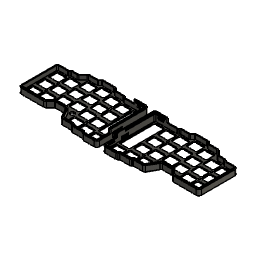
mriya-bumper-fdm-v1.04 (Autodesk Fusion 360 design; units mm, degrees)
Autodesk Fusion 360 part; units mm, degrees
(part 1 of 2)
sketch "mriya" plane through (0, 0, 0) normal (0, 0, 1) x (1, 0, 0)
  line L0 (-101.0213, 15.6719) -> (-94.7787, 21.9145) construction
  line L1 (-26.4858, 1.079) -> (-27.6142, 2.2074) construction
  line L2 (-138.1, 14.7932) -> (-103.1426, 14.7932) construction
  line L3 (-44.0716, 2.7932) -> (-29.0284, 2.7932) construction
  line L4 (-8.6, 0.4932) -> (-25.0716, 0.4932) construction
  line L5 (-64.4741, 6.1094) -> (-72.7517, 20.7608) construction
  line L6 (-45.4858, 3.379) -> (-46.6142, 4.5074) construction
  line L7 (-122.6142, 71.579) -> (-121.4858, 72.7074) construction
  line L8 (-101.0716, 81.2932) -> (-87.2284, 81.2932) construction
  line L9 (-138.1, 70.9932) -> (-124.0284, 70.9932) construction
  line L10 (-92.6574, 22.7932) -> (-76.2344, 22.7932) construction
  line L11 (-48.0284, 5.0932) -> (-62.7328, 5.0932) construction
  line L12 (-82.0716, 84.7932) -> (-64.7284, 84.7932) construction
  line L13 (-58.5716, 80.2932) -> (-45.7284, 80.2932) construction
  line L14 (-24.1, 19.4932) -> (-7.1, 19.4932) construction
  line L15 (-25.6, 20.9932) -> (-25.6, 77.9932) construction
  line L16 (-83.4858, 84.2074) -> (-85.8142, 81.879) construction
  line L17 (-63.3142, 84.2074) -> (-59.9858, 80.879) construction
  line L18 (-139.6, 69.4932) -> (-139.6, 16.2932) construction
  line L19 (-43.1858, 78.579) -> (-44.3142, 79.7074) construction
  line L20 (-99.4, 40.3932) -> (-99.4, 27.9932) construction
  line L21 (-98.6, 41.1932) -> (-86.2, 41.1932) construction
  line L22 (-98.6, 27.1932) -> (-86.2, 27.1932) construction
  line L23 (-85.4, 40.3932) -> (-85.4, 27.9932) construction
  line L24 (-42.4, 56.0932) -> (-42.4, 43.6932) construction
  line L25 (-41.6, 56.8932) -> (-29.2, 56.8932) construction
  line L26 (-41.6, 42.8932) -> (-29.2, 42.8932) construction
  line L27 (-28.4, 56.0932) -> (-28.4, 43.6932) construction
  line L28 (-61.4, 58.3932) -> (-61.4, 45.9932) construction
  line L29 (-60.6, 59.1932) -> (-48.2, 59.1932) construction
  line L30 (-60.6, 45.1932) -> (-48.2, 45.1932) construction
  line L31 (-47.4, 58.3932) -> (-47.4, 45.9932) construction
  line L32 (-137.4, 68.0932) -> (-137.4, 55.6932) construction
  line L33 (-136.6, 68.8932) -> (-124.2, 68.8932) construction
  line L34 (-136.6, 54.8932) -> (-124.2, 54.8932) construction
  line L35 (-123.4, 68.0932) -> (-123.4, 55.6932) construction
  line L36 (-61.4, 39.3932) -> (-61.4, 26.9932) construction
  line L37 (-60.6, 40.1932) -> (-48.2, 40.1932) construction
  line L38 (-60.6, 26.1932) -> (-48.2, 26.1932) construction
  line L39 (-47.4, 39.3932) -> (-47.4, 26.9932) construction
  line L40 (-42.4, 18.0932) -> (-42.4, 5.6932) construction
  line L41 (-41.6, 18.8932) -> (-29.2, 18.8932) construction
  line L42 (-41.6, 4.8932) -> (-29.2, 4.8932) construction
  line L43 (-28.4, 18.0932) -> (-28.4, 5.6932) construction
  line L44 (-23.4, 15.7932) -> (-23.4, 3.3932) construction
  line L45 (-22.6, 16.5932) -> (-10.2, 16.5932) construction
  line L46 (-22.6, 2.5932) -> (-10.2, 2.5932) construction
  line L47 (-9.4, 15.7932) -> (-9.4, 3.3932) construction
  line L48 (-137.4, 49.0932) -> (-137.4, 36.6932) construction
  line L49 (-136.6, 49.8932) -> (-124.2, 49.8932) construction
  line L50 (-136.6, 35.8932) -> (-124.2, 35.8932) construction
  line L51 (-123.4, 49.0932) -> (-123.4, 36.6932) construction
  line L52 (-118.4, 51.3932) -> (-118.4, 38.9932) construction
  line L53 (-117.6, 52.1932) -> (-105.2, 52.1932) construction
  line L54 (-117.6, 38.1932) -> (-105.2, 38.1932) construction
  line L55 (-104.4, 51.3932) -> (-104.4, 38.9932) construction
  line L56 (-137.4, 30.0932) -> (-137.4, 17.6932) construction
  line L57 (-136.6, 30.8932) -> (-124.2, 30.8932) construction
  line L58 (-136.6, 16.8932) -> (-124.2, 16.8932) construction
  line L59 (-123.4, 30.0932) -> (-123.4, 17.6932) construction
  line L60 (-61.4, 20.3932) -> (-61.4, 7.9932) construction
  line L61 (-60.6, 21.1932) -> (-48.2, 21.1932) construction
  line L62 (-60.6, 7.1932) -> (-48.2, 7.1932) construction
  line L63 (-47.4, 20.3932) -> (-47.4, 7.9932) construction
  line L64 (-80.4, 43.8932) -> (-80.4, 31.4932) construction
  line L65 (-79.6, 44.6932) -> (-67.2, 44.6932) construction
  line L66 (-79.6, 30.6932) -> (-67.2, 30.6932) construction
  line L67 (-66.4, 43.8932) -> (-66.4, 31.4932) construction
  line L68 (-80.4, 81.8932) -> (-80.4, 69.4932) construction
  line L69 (-79.6, 82.6932) -> (-67.2, 82.6932) construction
  line L70 (-79.6, 68.6932) -> (-67.2, 68.6932) construction
  line L71 (-66.4, 81.8932) -> (-66.4, 69.4932) construction
  line L72 (-42.4, 37.0932) -> (-42.4, 24.6932) construction
  line L73 (-41.6, 37.8932) -> (-29.2, 37.8932) construction
  line L74 (-41.6, 23.8932) -> (-29.2, 23.8932) construction
  line L75 (-28.4, 37.0932) -> (-28.4, 24.6932) construction
  line L76 (-118.4, 32.3932) -> (-118.4, 19.9932) construction
  line L77 (-117.6, 33.1932) -> (-105.2, 33.1932) construction
  line L78 (-117.6, 19.1932) -> (-105.2, 19.1932) construction
  line L79 (-104.4, 32.3932) -> (-104.4, 19.9932) construction
  line L80 (-61.4, 77.3932) -> (-61.4, 64.9932) construction
  line L81 (-60.6, 78.1932) -> (-48.2, 78.1932) construction
  line L82 (-60.6, 64.1932) -> (-48.2, 64.1932) construction
  line L83 (-47.4, 77.3932) -> (-47.4, 64.9932) construction
  line L84 (-42.4, 75.0932) -> (-42.4, 62.6932) construction
  line L85 (-41.6, 75.8932) -> (-29.2, 75.8932) construction
  line L86 (-41.6, 61.8932) -> (-29.2, 61.8932) construction
  line L87 (-28.4, 75.0932) -> (-28.4, 62.6932) construction
  line L88 (-118.4, 70.3932) -> (-118.4, 57.9932) construction
  line L89 (-117.6, 71.1932) -> (-105.2, 71.1932) construction
  line L90 (-117.6, 57.1932) -> (-105.2, 57.1932) construction
  line L91 (-104.4, 70.3932) -> (-104.4, 57.9932) construction
  line L92 (-99.4, 59.3932) -> (-99.4, 46.9932) construction
  line L93 (-98.6, 60.1932) -> (-86.2, 60.1932) construction
  line L94 (-98.6, 46.1932) -> (-86.2, 46.1932) construction
  line L95 (-85.4, 59.3932) -> (-85.4, 46.9932) construction
  line L96 (-80.4, 62.8932) -> (-80.4, 50.4932) construction
  line L97 (-79.6, 63.6932) -> (-67.2, 63.6932) construction
  line L98 (-79.6, 49.6932) -> (-67.2, 49.6932) construction
  line L99 (-66.4, 62.8932) -> (-66.4, 50.4932) construction
  line L100 (-99.4, 78.3932) -> (-99.4, 65.9932) construction
  line L101 (-98.6, 79.1932) -> (-86.2, 79.1932) construction
  line L102 (-98.6, 65.1932) -> (-86.2, 65.1932) construction
  line L103 (-85.4, 78.3932) -> (-85.4, 65.9932) construction
  circle A0 centre (-120.9, 53.5432) radius 1.6
  circle A1 centre (-120.9, 34.5432) radius 1.6
  circle A2 centre (-68.5, 23.5932) radius 3.5
  circle A3 centre (-44.9, 22.5432) radius 1.6
  circle A4 centre (-44.9, 60.5432) radius 1.6
  arc A5 (-43.1858, 78.579) -> (-41.7716, 77.9932) centre (-41.7716, 79.9932) ccw construction
  arc A6 (-44.3142, 79.7074) -> (-45.7284, 80.2932) centre (-45.7285, 78.2931) ccw construction
  arc A7 (-59.9858, 80.879) -> (-58.5716, 80.2932) centre (-58.5716, 82.2931) ccw construction
  arc A8 (-63.3142, 84.2074) -> (-64.7284, 84.7932) centre (-64.7285, 82.7931) ccw construction
  arc A9 (-82.0716, 84.7932) -> (-83.4858, 84.2074) centre (-82.0716, 82.7933) ccw construction
  arc A10 (-87.2284, 81.2932) -> (-85.8142, 81.879) centre (-87.2284, 83.2932) ccw construction
  arc A11 (-101.0716, 81.2932) -> (-102.4858, 80.7074) centre (-101.0716, 79.2933) ccw construction
  arc A12 (-120.0716, 73.2932) -> (-121.4858, 72.7074) centre (-120.0716, 71.2933) ccw construction
  arc A13 (-124.0284, 70.9932) -> (-122.6142, 71.579) centre (-124.0284, 72.9932) ccw construction
  arc A14 (-138.1, 70.9932) -> (-139.6, 69.4932) centre (-138.1, 69.4932) ccw construction
  arc A15 (-139.6, 16.2932) -> (-138.1, 14.7932) centre (-138.1, 16.2932) ccw construction
  arc A16 (-103.1426, 14.7932) -> (-101.0213, 15.6719) centre (-103.1426, 17.7931) ccw construction
  arc A17 (-92.6574, 22.7932) -> (-94.7787, 21.9145) centre (-92.6573, 19.7931) ccw construction
  arc A18 (-72.7517, 20.7608) -> (-76.2344, 22.7932) centre (-76.2344, 18.793) ccw construction
  arc A19 (-64.4741, 6.1094) -> (-62.7328, 5.0932) centre (-62.7328, 7.0932) ccw construction
  arc A20 (-46.6142, 4.5074) -> (-48.0284, 5.0932) centre (-48.0284, 3.0933) ccw construction
  arc A21 (-45.4858, 3.379) -> (-44.0716, 2.7932) centre (-44.0715, 4.7933) ccw construction
  arc A22 (-27.6142, 2.2074) -> (-29.0284, 2.7932) centre (-29.0284, 0.7933) ccw construction
  arc A23 (-26.4858, 1.079) -> (-25.0716, 0.4932) centre (-25.0715, 2.4933) ccw construction
  arc A24 (-8.6, 0.4932) -> (-7.1, 1.9932) centre (-8.6, 1.9932) ccw construction
  arc A25 (-25.6, 20.9932) -> (-24.1, 19.4932) centre (-24.1, 20.9932) ccw construction
  line L104 (-7.1, 1.9932) -> (-7.1, 76.4932) construction
  line L105 (-41.7716, 77.9932) -> (-8.6, 77.9932) construction
  arc A26 (-7.1, 76.4932) -> (-8.6, 77.9932) centre (-8.6, 76.4932) ccw construction
  arc A27 (-136.6, 68.8932) -> (-137.4, 68.0932) centre (-136.6, 68.0932) ccw construction
  arc A28 (-123.4, 68.0932) -> (-124.2, 68.8932) centre (-124.2, 68.0932) ccw construction
  arc A29 (-124.2, 54.8932) -> (-123.4, 55.6932) centre (-124.2, 55.6932) ccw construction
  arc A30 (-137.4, 55.6932) -> (-136.6, 54.8932) centre (-136.6, 55.6932) ccw construction
  arc A31 (-136.6, 49.8932) -> (-137.4, 49.0932) centre (-136.6, 49.0932) ccw construction
  arc A32 (-123.4, 49.0932) -> (-124.2, 49.8932) centre (-124.2, 49.0932) ccw construction
  arc A33 (-124.2, 35.8932) -> (-123.4, 36.6932) centre (-124.2, 36.6932) ccw construction
  arc A34 (-137.4, 36.6932) -> (-136.6, 35.8932) centre (-136.6, 36.6932) ccw construction
  arc A35 (-136.6, 30.8932) -> (-137.4, 30.0932) centre (-136.6, 30.0932) ccw construction
  arc A36 (-123.4, 30.0932) -> (-124.2, 30.8932) centre (-124.2, 30.0932) ccw construction
  arc A37 (-124.2, 16.8932) -> (-123.4, 17.6932) centre (-124.2, 17.6932) ccw construction
  arc A38 (-137.4, 17.6932) -> (-136.6, 16.8932) centre (-136.6, 17.6932) ccw construction
  arc A39 (-118.4, 19.9932) -> (-117.6, 19.1932) centre (-117.6, 19.9932) ccw construction
  arc A40 (-105.2, 19.1932) -> (-104.4, 19.9932) centre (-105.2, 19.9932) ccw construction
  arc A41 (-104.4, 32.3932) -> (-105.2, 33.1932) centre (-105.2, 32.3932) ccw construction
  arc A42 (-117.6, 33.1932) -> (-118.4, 32.3932) centre (-117.6, 32.3932) ccw construction
  arc A43 (-105.2, 38.1932) -> (-104.4, 38.9932) centre (-105.2, 38.9932) ccw construction
  arc A44 (-118.4, 38.9932) -> (-117.6, 38.1932) centre (-117.6, 38.9932) ccw construction
  arc A45 (-117.6, 52.1932) -> (-118.4, 51.3932) centre (-117.6, 51.3932) ccw construction
  arc A46 (-104.4, 51.3932) -> (-105.2, 52.1932) centre (-105.2, 51.3932) ccw construction
  arc A47 (-118.4, 57.9932) -> (-117.6, 57.1932) centre (-117.6, 57.9932) ccw construction
  arc A48 (-105.2, 57.1932) -> (-104.4, 57.9932) centre (-105.2, 57.9932) ccw construction
  arc A49 (-104.4, 70.3932) -> (-105.2, 71.1932) centre (-105.2, 70.3932) ccw construction
  arc A50 (-117.6, 71.1932) -> (-118.4, 70.3932) centre (-117.6, 70.3932) ccw construction
  arc A51 (-98.6, 79.1932) -> (-99.4, 78.3932) centre (-98.6, 78.3932) ccw construction
  arc A52 (-85.4, 78.3932) -> (-86.2, 79.1932) centre (-86.2, 78.3932) ccw construction
  arc A53 (-86.2, 65.1932) -> (-85.4, 65.9932) centre (-86.2, 65.9932) ccw construction
  arc A54 (-99.4, 65.9932) -> (-98.6, 65.1932) centre (-98.6, 65.9932) ccw construction
  arc A55 (-98.6, 60.1932) -> (-99.4, 59.3932) centre (-98.6, 59.3932) ccw construction
  arc A56 (-85.4, 59.3932) -> (-86.2, 60.1932) centre (-86.2, 59.3932) ccw construction
  arc A57 (-86.2, 46.1932) -> (-85.4, 46.9932) centre (-86.2, 46.9932) ccw construction
  arc A58 (-99.4, 46.9932) -> (-98.6, 46.1932) centre (-98.6, 46.9932) ccw construction
  arc A59 (-98.6, 41.1932) -> (-99.4, 40.3932) centre (-98.6, 40.3932) ccw construction
  arc A60 (-99.4, 27.9932) -> (-98.6, 27.1932) centre (-98.6, 27.9932) ccw construction
  arc A61 (-86.2, 27.1932) -> (-85.4, 27.9932) centre (-86.2, 27.9932) ccw construction
  arc A62 (-85.4, 40.3932) -> (-86.2, 41.1932) centre (-86.2, 40.3932) ccw construction
  arc A63 (-80.4, 31.4932) -> (-79.6, 30.6932) centre (-79.6, 31.4932) ccw construction
  arc A64 (-79.6, 44.6932) -> (-80.4, 43.8932) centre (-79.6, 43.8932) ccw construction
  arc A65 (-66.4, 43.8932) -> (-67.2, 44.6932) centre (-67.2, 43.8932) ccw construction
  arc A66 (-67.2, 30.6932) -> (-66.4, 31.4932) centre (-67.2, 31.4932) ccw construction
  arc A67 (-67.2, 49.6932) -> (-66.4, 50.4932) centre (-67.2, 50.4932) ccw construction
  arc A68 (-80.4, 50.4932) -> (-79.6, 49.6932) centre (-79.6, 50.4932) ccw construction
  arc A69 (-79.6, 63.6932) -> (-80.4, 62.8932) centre (-79.6, 62.8932) ccw construction
  arc A70 (-66.4, 62.8932) -> (-67.2, 63.6932) centre (-67.2, 62.8932) ccw construction
  arc A71 (-67.2, 68.6932) -> (-66.4, 69.4932) centre (-67.2, 69.4932) ccw construction
  arc A72 (-80.4, 69.4932) -> (-79.6, 68.6932) centre (-79.6, 69.4932) ccw construction
  arc A73 (-79.6, 82.6932) -> (-80.4, 81.8932) centre (-79.6, 81.8932) ccw construction
  arc A74 (-66.4, 81.8932) -> (-67.2, 82.6932) centre (-67.2, 81.8932) ccw construction
  arc A75 (-60.6, 78.1932) -> (-61.4, 77.3932) centre (-60.6, 77.3932) ccw construction
  arc A76 (-61.4, 64.9932) -> (-60.6, 64.1932) centre (-60.6, 64.9932) ccw construction
  arc A77 (-48.2, 64.1932) -> (-47.4, 64.9932) centre (-48.2, 64.9932) ccw construction
  arc A78 (-47.4, 77.3932) -> (-48.2, 78.1932) centre (-48.2, 77.3932) ccw construction
  arc A79 (-47.4, 58.3932) -> (-48.2, 59.1932) centre (-48.2, 58.3932) ccw construction
  arc A80 (-60.6, 59.1932) -> (-61.4, 58.3932) centre (-60.6, 58.3932) ccw construction
  arc A81 (-61.4, 45.9932) -> (-60.6, 45.1932) centre (-60.6, 45.9932) ccw construction
  arc A82 (-48.2, 45.1932) -> (-47.4, 45.9932) centre (-48.2, 45.9932) ccw construction
  arc A83 (-47.4, 39.3932) -> (-48.2, 40.1932) centre (-48.2, 39.3932) ccw construction
  arc A84 (-60.6, 40.1932) -> (-61.4, 39.3932) centre (-60.6, 39.3932) ccw construction
  arc A85 (-61.4, 26.9932) -> (-60.6, 26.1932) centre (-60.6, 26.9932) ccw construction
  arc A86 (-48.2, 26.1932) -> (-47.4, 26.9932) centre (-48.2, 26.9932) ccw construction
  arc A87 (-47.4, 20.3932) -> (-48.2, 21.1932) centre (-48.2, 20.3932) ccw construction
  arc A88 (-60.6, 21.1932) -> (-61.4, 20.3932) centre (-60.6, 20.3932) ccw construction
  arc A89 (-61.4, 7.9932) -> (-60.6, 7.1932) centre (-60.6, 7.9932) ccw construction
  arc A90 (-48.2, 7.1932) -> (-47.4, 7.9932) centre (-48.2, 7.9932) ccw construction
  arc A91 (-42.4, 5.6932) -> (-41.6, 4.8932) centre (-41.6, 5.6932) ccw construction
  arc A92 (-29.2, 4.8932) -> (-28.4, 5.6932) centre (-29.2, 5.6932) ccw construction
  arc A93 (-28.4, 18.0932) -> (-29.2, 18.8932) centre (-29.2, 18.0932) ccw construction
  arc A94 (-41.6, 18.8932) -> (-42.4, 18.0932) centre (-41.6, 18.0932) ccw construction
  arc A95 (-23.4, 3.3932) -> (-22.6, 2.5932) centre (-22.6, 3.3932) ccw construction
  arc A96 (-10.2, 2.5932) -> (-9.4, 3.3932) centre (-10.2, 3.3932) ccw construction
  arc A97 (-9.4, 15.7932) -> (-10.2, 16.5932) centre (-10.2, 15.7932) ccw construction
  arc A98 (-22.6, 16.5932) -> (-23.4, 15.7932) centre (-22.6, 15.7932) ccw construction
  arc A99 (-29.2, 23.8932) -> (-28.4, 24.6932) centre (-29.2, 24.6932) ccw construction
  arc A100 (-42.4, 24.6932) -> (-41.6, 23.8932) centre (-41.6, 24.6932) ccw construction
  arc A101 (-41.6, 37.8932) -> (-42.4, 37.0932) centre (-41.6, 37.0932) ccw construction
  arc A102 (-28.4, 37.0932) -> (-29.2, 37.8932) centre (-29.2, 37.0932) ccw construction
  arc A103 (-29.2, 42.8932) -> (-28.4, 43.6932) centre (-29.2, 43.6932) ccw construction
  arc A104 (-42.4, 43.6932) -> (-41.6, 42.8932) centre (-41.6, 43.6932) ccw construction
  arc A105 (-41.6, 56.8932) -> (-42.4, 56.0932) centre (-41.6, 56.0932) ccw construction
  arc A106 (-28.4, 56.0932) -> (-29.2, 56.8932) centre (-29.2, 56.0932) ccw construction
  arc A107 (-29.2, 61.8932) -> (-28.4, 62.6932) centre (-29.2, 62.6932) ccw construction
  arc A108 (-42.4, 62.6932) -> (-41.6, 61.8932) centre (-41.6, 62.6932) ccw construction
  arc A109 (-41.6, 75.8932) -> (-42.4, 75.0932) centre (-41.6, 75.0932) ccw construction
  arc A110 (-28.4, 75.0932) -> (-29.2, 75.8932) centre (-29.2, 75.0932) ccw construction
  circle A111 centre (-22.6, 22.4932) radius 1.1 construction
  circle A112 centre (-10.2, 22.4932) radius 1.1 construction
  line L106 (-23.6, 77.8432) -> (-23.6, 78.1432)
  line L107 (-23, 77.2432) -> (-8.65, 77.2432)
  line L108 (-7.85, 32.0932) -> (-7.85, 76.4432)
  arc A113 (-7.85, 76.4432) -> (-8.65, 77.2432) centre (-8.65, 76.4432) ccw
  arc A114 (-23.6, 77.8432) -> (-23, 77.2432) centre (-23, 77.8432) ccw
  arc A115 (-7.85, 32.0932) -> (-7.25, 31.4932) centre (-7.25, 32.0932) ccw
  line L109 (-6.95, 14.5932) -> (-7.25, 14.5932)
  line L110 (-7.85, 13.9932) -> (-7.85, 5.1932)
  arc A116 (-7.25, 14.5932) -> (-7.85, 13.9932) centre (-7.25, 13.9932) ccw
  arc A117 (-7.85, 5.1932) -> (-7.25, 4.5932) centre (-7.25, 5.1932) ccw
  line L111 (-102.4858, 80.7074) -> (-109.0213, 74.1719) construction
  line L112 (-120.0716, 73.2932) -> (-111.1426, 73.2932) construction
  arc A118 (-111.1426, 73.2932) -> (-109.0213, 74.1719) centre (-111.1426, 76.2932) ccw construction
  arc A119 (-64.7284, 82.7932) -> (-64.7285, 82.7932) centre (-64.7285, 82.7931) ccw
  arc A120 (-45.7284, 78.2932) -> (-45.7285, 78.2932) centre (-45.7285, 78.2931) ccw
  arc A121 (-25.0716, 2.4932) -> (-25.0715, 2.4932) centre (-25.0715, 2.4933) ccw
  arc A122 (-44.0716, 4.7932) -> (-44.0715, 4.7932) centre (-44.0715, 4.7933) ccw
  line L113 (-123.9, 54.8932) -> (-136.9, 54.8932)
  line L114 (-138.9, 56.8932) -> (-138.9, 66.8932)
  line L115 (-136.9, 68.8932) -> (-123.9, 68.8932)
  line L116 (-121.9, 66.8932) -> (-121.9, 56.8932)
  arc A123 (-121.9, 66.8932) -> (-123.9, 68.8932) centre (-123.9, 66.8932) ccw
  arc A124 (-123.9, 54.8932) -> (-121.9, 56.8932) centre (-123.9, 56.8932) ccw
  arc A125 (-138.9, 56.8932) -> (-136.9, 54.8932) centre (-136.9, 56.8932) ccw
  arc A126 (-136.9, 68.8932) -> (-138.9, 66.8932) centre (-136.9, 66.8932) ccw
  arc A127 (-123.9, 35.8932) -> (-121.9, 37.8932) centre (-123.9, 37.8932) ccw
  line L117 (-123.9, 35.8932) -> (-136.9, 35.8932)
  arc A128 (-138.9, 37.8932) -> (-136.9, 35.8932) centre (-136.9, 37.8932) ccw
  line L118 (-138.9, 37.8932) -> (-138.9, 47.8932)
  arc A129 (-136.9, 49.8932) -> (-138.9, 47.8932) centre (-136.9, 47.8932) ccw
  line L119 (-136.9, 49.8932) -> (-123.9, 49.8932)
  arc A130 (-121.9, 47.8932) -> (-123.9, 49.8932) centre (-123.9, 47.8932) ccw
  line L120 (-121.9, 47.8932) -> (-121.9, 37.8932)
  arc A131 (-123.9, 16.8932) -> (-121.9, 18.8932) centre (-123.9, 18.8932) ccw
  line L121 (-123.9, 16.8932) -> (-136.9, 16.8932)
  arc A132 (-138.9, 18.8932) -> (-136.9, 16.8932) centre (-136.9, 18.8932) ccw
  line L122 (-138.9, 18.8932) -> (-138.9, 28.8932)
  arc A133 (-136.9, 30.8932) -> (-138.9, 28.8932) centre (-136.9, 28.8932) ccw
  line L123 (-136.9, 30.8932) -> (-123.9, 30.8932)
  arc A134 (-121.9, 28.8932) -> (-123.9, 30.8932) centre (-123.9, 28.8932) ccw
  line L124 (-121.9, 28.8932) -> (-121.9, 18.8932)
  arc A135 (-104.9, 57.1932) -> (-102.9, 59.1932) centre (-104.9, 59.1932) ccw
  line L125 (-104.9, 57.1932) -> (-117.9, 57.1932)
  arc A136 (-119.9, 59.1932) -> (-117.9, 57.1932) centre (-117.9, 59.1932) ccw
  line L126 (-119.9, 59.1932) -> (-119.9, 69.1932)
  arc A137 (-117.9, 71.1932) -> (-119.9, 69.1932) centre (-117.9, 69.1932) ccw
  line L127 (-117.9, 71.1932) -> (-104.9, 71.1932)
  arc A138 (-102.9, 69.1932) -> (-104.9, 71.1932) centre (-104.9, 69.1932) ccw
  line L128 (-102.9, 69.1932) -> (-102.9, 59.1932)
  arc A139 (-104.9, 38.1932) -> (-102.9, 40.1932) centre (-104.9, 40.1932) ccw
  line L129 (-104.9, 38.1932) -> (-117.9, 38.1932)
  arc A140 (-119.9, 40.1932) -> (-117.9, 38.1932) centre (-117.9, 40.1932) ccw
  line L130 (-119.9, 40.1932) -> (-119.9, 50.1932)
  arc A141 (-117.9, 52.1932) -> (-119.9, 50.1932) centre (-117.9, 50.1932) ccw
  line L131 (-117.9, 52.1932) -> (-104.9, 52.1932)
  arc A142 (-102.9, 50.1932) -> (-104.9, 52.1932) centre (-104.9, 50.1932) ccw
  line L132 (-102.9, 50.1932) -> (-102.9, 40.1932)
  arc A143 (-104.9, 19.1932) -> (-102.9, 21.1932) centre (-104.9, 21.1932) ccw
  line L133 (-104.9, 19.1932) -> (-117.9, 19.1932)
  arc A144 (-119.9, 21.1932) -> (-117.9, 19.1932) centre (-117.9, 21.1932) ccw
  line L134 (-119.9, 21.1932) -> (-119.9, 31.1932)
  arc A145 (-117.9, 33.1932) -> (-119.9, 31.1932) centre (-117.9, 31.1932) ccw
  line L135 (-117.9, 33.1932) -> (-104.9, 33.1932)
  arc A146 (-102.9, 31.1932) -> (-104.9, 33.1932) centre (-104.9, 31.1932) ccw
  line L136 (-102.9, 31.1932) -> (-102.9, 21.1932)
  arc A147 (-85.9, 65.1932) -> (-83.9, 67.1932) centre (-85.9, 67.1932) ccw
  line L137 (-85.9, 65.1932) -> (-98.9, 65.1932)
  arc A148 (-100.9, 67.1932) -> (-98.9, 65.1932) centre (-98.9, 67.1932) ccw
  line L138 (-100.9, 67.1932) -> (-100.9, 77.1932)
  arc A149 (-98.9, 79.1932) -> (-100.9, 77.1932) centre (-98.9, 77.1932) ccw
  line L139 (-98.9, 79.1932) -> (-85.9, 79.1932)
  arc A150 (-83.9, 77.1932) -> (-85.9, 79.1932) centre (-85.9, 77.1932) ccw
  line L140 (-83.9, 77.1932) -> (-83.9, 67.1932)
  arc A151 (-85.9, 46.1932) -> (-83.9, 48.1932) centre (-85.9, 48.1932) ccw
  line L141 (-85.9, 46.1932) -> (-98.9, 46.1932)
  arc A152 (-100.9, 48.1932) -> (-98.9, 46.1932) centre (-98.9, 48.1932) ccw
  line L142 (-100.9, 48.1932) -> (-100.9, 58.1932)
  arc A153 (-98.9, 60.1932) -> (-100.9, 58.1932) centre (-98.9, 58.1932) ccw
  line L143 (-98.9, 60.1932) -> (-85.9, 60.1932)
  arc A154 (-83.9, 58.1932) -> (-85.9, 60.1932) centre (-85.9, 58.1932) ccw
  line L144 (-83.9, 58.1932) -> (-83.9, 48.1932)
  arc A155 (-85.9, 27.1932) -> (-83.9, 29.1932) centre (-85.9, 29.1932) ccw
  line L145 (-85.9, 27.1932) -> (-98.9, 27.1932)
  arc A156 (-100.9, 29.1932) -> (-98.9, 27.1932) centre (-98.9, 29.1932) ccw
  line L146 (-100.9, 29.1932) -> (-100.9, 39.1932)
  arc A157 (-98.9, 41.1932) -> (-100.9, 39.1932) centre (-98.9, 39.1932) ccw
  line L147 (-98.9, 41.1932) -> (-85.9, 41.1932)
  arc A158 (-83.9, 39.1932) -> (-85.9, 41.1932) centre (-85.9, 39.1932) ccw
  line L148 (-83.9, 39.1932) -> (-83.9, 29.1932)
  arc A159 (-66.9, 30.6932) -> (-64.9, 32.6932) centre (-66.9, 32.6932) ccw
  line L149 (-66.9, 30.6932) -> (-79.9, 30.6932)
  arc A160 (-81.9, 32.6932) -> (-79.9, 30.6932) centre (-79.9, 32.6932) ccw
  line L150 (-81.9, 32.6932) -> (-81.9, 42.6932)
  arc A161 (-79.9, 44.6932) -> (-81.9, 42.6932) centre (-79.9, 42.6932) ccw
  line L151 (-79.9, 44.6932) -> (-66.9, 44.6932)
  arc A162 (-64.9, 42.6932) -> (-66.9, 44.6932) centre (-66.9, 42.6932) ccw
  line L152 (-64.9, 42.6932) -> (-64.9, 32.6932)
  arc A163 (-66.9, 49.6932) -> (-64.9, 51.6932) centre (-66.9, 51.6932) ccw
  line L153 (-66.9, 49.6932) -> (-79.9, 49.6932)
  arc A164 (-81.9, 51.6932) -> (-79.9, 49.6932) centre (-79.9, 51.6932) ccw
  line L154 (-81.9, 51.6932) -> (-81.9, 61.6932)
  arc A165 (-79.9, 63.6932) -> (-81.9, 61.6932) centre (-79.9, 61.6932) ccw
  line L155 (-79.9, 63.6932) -> (-66.9, 63.6932)
  arc A166 (-64.9, 61.6932) -> (-66.9, 63.6932) centre (-66.9, 61.6932) ccw
  line L156 (-64.9, 61.6932) -> (-64.9, 51.6932)
  arc A167 (-66.9, 68.6932) -> (-64.9, 70.6932) centre (-66.9, 70.6932) ccw
  line L157 (-66.9, 68.6932) -> (-79.9, 68.6932)
  arc A168 (-81.9, 70.6932) -> (-79.9, 68.6932) centre (-79.9, 70.6932) ccw
  line L158 (-81.9, 70.6932) -> (-81.9, 80.6932)
  arc A169 (-79.9, 82.6932) -> (-81.9, 80.6932) centre (-79.9, 80.6932) ccw
  line L159 (-79.9, 82.6932) -> (-66.9, 82.6932)
  arc A170 (-64.9, 80.6932) -> (-66.9, 82.6932) centre (-66.9, 80.6932) ccw
  line L160 (-64.9, 80.6932) -> (-64.9, 70.6932)
  arc A171 (-47.9, 26.1932) -> (-45.9, 28.1932) centre (-47.9, 28.1932) ccw
  line L161 (-47.9, 26.1932) -> (-60.9, 26.1932)
  arc A172 (-62.9, 28.1932) -> (-60.9, 26.1932) centre (-60.9, 28.1932) ccw
  line L162 (-62.9, 28.1932) -> (-62.9, 38.1932)
  arc A173 (-60.9, 40.1932) -> (-62.9, 38.1932) centre (-60.9, 38.1932) ccw
  line L163 (-60.9, 40.1932) -> (-47.9, 40.1932)
  arc A174 (-45.9, 38.1932) -> (-47.9, 40.1932) centre (-47.9, 38.1932) ccw
  line L164 (-45.9, 38.1932) -> (-45.9, 28.1932)
  arc A175 (-47.9, 45.1932) -> (-45.9, 47.1932) centre (-47.9, 47.1932) ccw
  line L165 (-47.9, 45.1932) -> (-60.9, 45.1932)
  arc A176 (-62.9, 47.1932) -> (-60.9, 45.1932) centre (-60.9, 47.1932) ccw
  line L166 (-62.9, 47.1932) -> (-62.9, 57.1932)
  arc A177 (-60.9, 59.1932) -> (-62.9, 57.1932) centre (-60.9, 57.1932) ccw
  line L167 (-60.9, 59.1932) -> (-47.9, 59.1932)
  arc A178 (-45.9, 57.1932) -> (-47.9, 59.1932) centre (-47.9, 57.1932) ccw
  line L168 (-45.9, 57.1932) -> (-45.9, 47.1932)
  arc A179 (-47.9, 64.1932) -> (-45.9, 66.1932) centre (-47.9, 66.1932) ccw
  line L169 (-47.9, 64.1932) -> (-60.9, 64.1932)
  arc A180 (-62.9, 66.1932) -> (-60.9, 64.1932) centre (-60.9, 66.1932) ccw
  line L170 (-62.9, 66.1932) -> (-62.9, 76.1932)
  arc A181 (-60.9, 78.1932) -> (-62.9, 76.1932) centre (-60.9, 76.1932) ccw
  line L171 (-60.9, 78.1932) -> (-47.9, 78.1932)
  arc A182 (-45.9, 76.1932) -> (-47.9, 78.1932) centre (-47.9, 76.1932) ccw
  line L172 (-45.9, 76.1932) -> (-45.9, 66.1932)
  arc A183 (-47.9, 7.1932) -> (-45.9, 9.1932) centre (-47.9, 9.1932) ccw
  line L173 (-47.9, 7.1932) -> (-60.9, 7.1932)
  arc A184 (-62.9, 9.1932) -> (-60.9, 7.1932) centre (-60.9, 9.1932) ccw
  line L174 (-62.9, 9.1932) -> (-62.9, 19.1932)
  arc A185 (-60.9, 21.1932) -> (-62.9, 19.1932) centre (-60.9, 19.1932) ccw
  line L175 (-60.9, 21.1932) -> (-47.9, 21.1932)
  arc A186 (-45.9, 19.1932) -> (-47.9, 21.1932) centre (-47.9, 19.1932) ccw
  line L176 (-45.9, 19.1932) -> (-45.9, 9.1932)
  arc A187 (-28.9, 4.8932) -> (-26.9, 6.8932) centre (-28.9, 6.8932) ccw
  line L177 (-28.9, 4.8932) -> (-41.9, 4.8932)
  arc A188 (-43.9, 6.8932) -> (-41.9, 4.8932) centre (-41.9, 6.8932) ccw
  line L178 (-43.9, 6.8932) -> (-43.9, 16.8932)
  arc A189 (-41.9, 18.8932) -> (-43.9, 16.8932) centre (-41.9, 16.8932) ccw
  line L179 (-41.9, 18.8932) -> (-28.9, 18.8932)
  arc A190 (-26.9, 16.8932) -> (-28.9, 18.8932) centre (-28.9, 16.8932) ccw
  line L180 (-26.9, 16.8932) -> (-26.9, 6.8932)
  arc A191 (-28.9, 23.8932) -> (-26.9, 25.8932) centre (-28.9, 25.8932) ccw
  line L181 (-28.9, 23.8932) -> (-41.9, 23.8932)
  arc A192 (-43.9, 25.8932) -> (-41.9, 23.8932) centre (-41.9, 25.8932) ccw
  line L182 (-43.9, 25.8932) -> (-43.9, 35.8932)
  arc A193 (-41.9, 37.8932) -> (-43.9, 35.8932) centre (-41.9, 35.8932) ccw
  line L183 (-41.9, 37.8932) -> (-28.9, 37.8932)
  arc A194 (-26.9, 35.8932) -> (-28.9, 37.8932) centre (-28.9, 35.8932) ccw
  line L184 (-26.9, 35.8932) -> (-26.9, 25.8932)
  arc A195 (-28.9, 42.8932) -> (-26.9, 44.8932) centre (-28.9, 44.8932) ccw
  line L185 (-28.9, 42.8932) -> (-41.9, 42.8932)
  arc A196 (-43.9, 44.8932) -> (-41.9, 42.8932) centre (-41.9, 44.8932) ccw
  line L186 (-43.9, 44.8932) -> (-43.9, 54.8932)
  arc A197 (-41.9, 56.8932) -> (-43.9, 54.8932) centre (-41.9, 54.8932) ccw
  line L187 (-41.9, 56.8932) -> (-28.9, 56.8932)
  arc A198 (-26.9, 54.8932) -> (-28.9, 56.8932) centre (-28.9, 54.8932) ccw
  line L188 (-26.9, 54.8932) -> (-26.9, 44.8932)
  arc A199 (-28.9, 61.8932) -> (-26.9, 63.8932) centre (-28.9, 63.8932) ccw
  line L189 (-28.9, 61.8932) -> (-41.9, 61.8932)
  arc A200 (-43.9, 63.8932) -> (-41.9, 61.8932) centre (-41.9, 63.8932) ccw
  line L190 (-43.9, 63.8932) -> (-43.9, 73.8932)
  arc A201 (-41.9, 75.8932) -> (-43.9, 73.8932) centre (-41.9, 73.8932) ccw
  line L191 (-41.9, 75.8932) -> (-28.9, 75.8932)
  arc A202 (-26.9, 73.8932) -> (-28.9, 75.8932) centre (-28.9, 73.8932) ccw
  line L192 (-26.9, 73.8932) -> (-26.9, 63.8932)
  arc A203 (-9.9, 2.5932) -> (-7.9, 4.5932) centre (-9.9, 4.5932) ccw
  line L193 (-9.9, 2.5932) -> (-22.9, 2.5932)
  arc A204 (-24.9, 4.5932) -> (-22.9, 2.5932) centre (-22.9, 4.5932) ccw
  line L194 (-24.9, 4.5932) -> (-24.9, 14.5932)
  arc A205 (-22.9, 16.5932) -> (-24.9, 14.5932) centre (-22.9, 14.5932) ccw
  line L195 (-22.9, 16.5932) -> (-9.9, 16.5932)
  arc A206 (-7.9, 14.5932) -> (-9.9, 16.5932) centre (-9.9, 14.5932) ccw
  line L196 (-7.9, 14.5932) -> (-7.9, 4.5932)
  arc A207 (-9.9, 19.8932) -> (-7.9, 21.8932) centre (-9.9, 21.8932) ccw
  line L197 (-9.9, 19.8932) -> (-22.9, 19.8932)
  arc A208 (-24.9, 21.8932) -> (-22.9, 19.8932) centre (-22.9, 21.8932) ccw
  line L198 (-24.9, 21.8932) -> (-24.9, 73.8932)
  arc A209 (-22.9, 75.8932) -> (-24.9, 73.8932) centre (-22.9, 73.8932) ccw
  line L199 (-22.9, 75.8932) -> (-9.9, 75.8932)
  arc A210 (-7.9, 73.8932) -> (-9.9, 75.8932) centre (-9.9, 73.8932) ccw
  line L200 (-7.9, 73.8932) -> (-7.9, 21.8932)
  line L201 (-102.5919, 80.8135) -> (-109.1274, 74.2779)
  arc A211 (-111.1426, 73.4432) -> (-109.1274, 74.2779) centre (-111.1426, 76.2932) ccw
  line L202 (-120.0716, 73.4432) -> (-111.1426, 73.4432)
  arc A212 (-120.0716, 73.4432) -> (-121.5919, 72.8135) centre (-120.0716, 71.2933) ccw
  line L203 (-122.7203, 71.6851) -> (-121.5919, 72.8135)
  arc A213 (-124.0284, 71.1432) -> (-122.7203, 71.6851) centre (-124.0284, 72.9932) ccw
  line L204 (-138.1, 71.1432) -> (-124.0284, 71.1432)
  arc A214 (-138.1, 71.1432) -> (-139.75, 69.4932) centre (-138.1, 69.4932) ccw
  line L205 (-139.75, 69.4932) -> (-139.75, 16.2932)
  arc A215 (-139.75, 16.2932) -> (-138.1, 14.6432) centre (-138.1, 16.2932) ccw
  line L206 (-138.1, 14.6432) -> (-103.1426, 14.6432)
  arc A216 (-103.1426, 14.6432) -> (-100.9152, 15.5658) centre (-103.1426, 17.7931) ccw
  line L207 (-100.9152, 15.5658) -> (-94.6726, 21.8084)
  arc A217 (-92.6574, 22.6432) -> (-94.6726, 21.8084) centre (-92.6573, 19.7931) ccw
  line L208 (-92.6574, 22.6432) -> (-76.2344, 22.6432)
  arc A218 (-72.8823, 20.687) -> (-76.2344, 22.6432) centre (-76.2344, 18.793) ccw
  line L209 (-64.6047, 6.0356) -> (-72.8823, 20.687)
  arc A219 (-64.6047, 6.0356) -> (-62.7328, 4.9432) centre (-62.7328, 7.0932) ccw
  line L210 (-48.0284, 4.9432) -> (-62.7328, 4.9432)
  arc A220 (-46.7203, 4.4013) -> (-48.0284, 4.9432) centre (-48.0284, 3.0933) ccw
  line L211 (-45.5919, 3.2729) -> (-46.7203, 4.4013)
  arc A221 (-45.5919, 3.2729) -> (-44.0716, 2.6432) centre (-44.0715, 4.7933) ccw
  line L212 (-44.0716, 2.6432) -> (-29.0284, 2.6432)
  arc A222 (-27.7203, 2.1013) -> (-29.0284, 2.6432) centre (-29.0284, 0.7933) ccw
  line L213 (-26.5919, 0.9729) -> (-27.7203, 2.1013)
  arc A223 (-26.5919, 0.9729) -> (-25.0716, 0.3432) centre (-25.0715, 2.4933) ccw
  line L214 (-8.6, 0.3432) -> (-25.0716, 0.3432)
  arc A224 (-8.6, 0.3432) -> (-6.95, 1.9932) centre (-8.6, 1.9932) ccw
  line L215 (-6.95, 1.9932) -> (-6.95, 76.4932)
  arc A225 (-6.95, 76.4932) -> (-8.6, 78.1432) centre (-8.6, 76.4932) ccw
  line L216 (-41.7716, 78.1432) -> (-8.6, 78.1432)
  arc A226 (-43.0797, 78.6851) -> (-41.7716, 78.1432) centre (-41.7716, 79.9932) ccw
  line L217 (-43.0797, 78.6851) -> (-44.2081, 79.8135)
  arc A227 (-44.2081, 79.8135) -> (-45.7284, 80.4432) centre (-45.7285, 78.2931) ccw
  line L218 (-58.5716, 80.4432) -> (-45.7284, 80.4432)
  arc A228 (-59.8797, 80.9851) -> (-58.5716, 80.4432) centre (-58.5716, 82.2931) ccw
  line L219 (-63.2081, 84.3135) -> (-59.8797, 80.9851)
  arc A229 (-63.2081, 84.3135) -> (-64.7284, 84.9432) centre (-64.7285, 82.7931) ccw
  line L220 (-82.0716, 84.9432) -> (-64.7284, 84.9432)
  arc A230 (-82.0716, 84.9432) -> (-83.5919, 84.3135) centre (-82.0716, 82.7933) ccw
  line L221 (-83.5919, 84.3135) -> (-85.9203, 81.9851)
  arc A231 (-87.2284, 81.4432) -> (-85.9203, 81.9851) centre (-87.2284, 83.2932) ccw
  line L222 (-101.0716, 81.4432) -> (-87.2284, 81.4432)
  arc A232 (-101.0716, 81.4432) -> (-102.5919, 80.8135) centre (-101.0716, 79.2933) ccw
  line L223 (-91.9739, 20.1432) -> (-77.1972, 20.1432)
  line L224 (-99.4844, 13.4608) -> (-93.3848, 19.5589)
  line L225 (-138.1, 12.1432) -> (-102.666, 12.1432)
  arc A233 (-142.25, 16.2932) -> (-138.1, 12.1432) centre (-138.1, 16.2932) ccw
  line L226 (-142.25, 69.4932) -> (-142.25, 16.2932)
  arc A234 (-138.1, 73.6432) -> (-142.25, 69.4932) centre (-138.1, 69.4932) ccw
  line L227 (-138.1, 73.6432) -> (-124.7119, 73.6432)
  line L228 (-124.0048, 73.9361) -> (-122.8763, 75.0645)
  line L229 (-120.755, 75.9432) -> (-111.619, 75.9432)
  line L230 (-103.8763, 83.0645) -> (-110.5583, 76.3825)
  line L231 (-101.755, 83.9432) -> (-87.9119, 83.9432)
  line L232 (-84.8763, 86.5645) -> (-87.2048, 84.2361)
  line L233 (-82.755, 87.4432) -> (-64.0453, 87.4432)
  line L234 (-61.9236, 86.5642) -> (-58.5977, 83.2372)
  line L235 (-57.8881, 82.9432) -> (-45.045, 82.9432)
  line L236 (-41.7952, 80.9361) -> (-42.9237, 82.0645)
  line L237 (-41.0881, 80.6432) -> (-8.6, 80.6432)
  arc A235 (-4.45, 76.4932) -> (-8.6, 80.6432) centre (-8.6, 76.4932) ccw
  line L238 (-4.45, 1.9932) -> (-4.45, 76.4932)
  arc A236 (-8.6, -2.1568) -> (-4.45, 1.9932) centre (-8.6, 1.9932) ccw
  line L239 (-8.6, -2.1568) -> (-25.7597, -2.1568)
  line L240 (-27.8754, -1.2837) -> (-29.0249, -0.1403)
  line L241 (-44.755, 0.1432) -> (-29.7119, 0.1432)
  line L242 (-46.8763, 1.0219) -> (-48.0048, 2.1503)
  line L243 (-48.7119, 2.4432) -> (-63.4039, 2.4432)
  line L244 (-66.4512, 4.2216) -> (-74.5853, 18.6189)
  arc A237 (-91.9739, 20.1432) -> (-93.3848, 19.5589) centre (-91.9739, 18.1477) ccw
  arc A238 (-74.5853, 18.6189) -> (-77.1972, 20.1432) centre (-77.1972, 17.1432) ccw
  arc A239 (-29.0249, -0.1403) -> (-29.7119, 0.1432) centre (-29.7119, -0.831) ccw
  arc A240 (-48.0048, 2.1503) -> (-48.7119, 2.4432) centre (-48.7119, 1.4432) ccw
  arc A241 (-66.4512, 4.2216) -> (-63.4039, 2.4432) centre (-63.4039, 5.9432) ccw
  arc A242 (-46.8763, 1.0219) -> (-44.755, 0.1432) centre (-44.755, 3.1432) ccw
  arc A243 (-27.8754, -1.2837) -> (-25.7597, -2.1568) centre (-25.7597, 0.8432) ccw
  arc A244 (-102.666, 12.1432) -> (-99.4844, 13.4608) centre (-102.666, 16.6432) ccw
  line L245 (-25.8, 78.1432) -> (-25.8, 80.6432)
  arc A245 (-124.7119, 73.6432) -> (-124.0048, 73.9361) centre (-124.7119, 74.6432) ccw
  arc A246 (-120.755, 75.9432) -> (-122.8763, 75.0645) centre (-120.755, 72.9432) ccw
  arc A247 (-111.619, 75.9432) -> (-110.5583, 76.3825) centre (-111.619, 77.4432) ccw
  arc A248 (-101.755, 83.9432) -> (-103.8763, 83.0645) centre (-101.755, 80.9432) ccw
  arc A249 (-87.9119, 83.9432) -> (-87.2048, 84.2361) centre (-87.9119, 84.9432) ccw
  arc A250 (-82.755, 87.4432) -> (-84.8763, 86.5645) centre (-82.755, 84.4432) ccw
  arc A251 (-58.5977, 83.2372) -> (-57.8881, 82.9432) centre (-57.8881, 83.9465) ccw
  arc A252 (-61.9236, 86.5642) -> (-64.0453, 87.4432) centre (-64.0453, 84.4432) ccw
  arc A253 (-41.7952, 80.9361) -> (-41.0881, 80.6432) centre (-41.0881, 81.6432) ccw
  arc A254 (-42.9237, 82.0645) -> (-45.045, 82.9432) centre (-45.045, 79.9432) ccw
  line L246 (-7.25, 31.4932) -> (-6.95, 31.4932)
  line L247 (-7.25, 4.5932) -> (-6.95, 4.5932)
  line L248 (-6.95, 19.2932) -> (-4.45, 19.2932)
  dimension "d1" = 3.2
  dimension "d2" = 3.2
  dimension "d3" = 7
  dimension "d4" = 3.2
  dimension "d5" = 3.2
  dimension "d9" = 2.2
  dimension "d12" = 2.2
  constraint tangent L19 A5
  constraint tangent L19 A6
  constraint tangent L13 A7
  constraint tangent L17 A8
  constraint tangent L12 A9
  constraint tangent L16 A10
  constraint tangent L8 A11
  constraint tangent L7 A13
  constraint tangent L9 A14
  constraint tangent L18 A15
  constraint tangent L2 A16
  constraint tangent L0 A17
  constraint tangent L10 A18
  constraint tangent L5 A19
  constraint tangent L11 A20
  constraint tangent L6 A21
  constraint tangent L3 A22
  constraint tangent L1 A23
  constraint tangent L4 A24
  constraint tangent L15 A25
  constraint tangent A24 L104
  constraint perpendicular L104 L105
  constraint tangent L104 A26
  constraint tangent L105 A26
  constraint coincident L15.end L105
  constraint perpendicular L15 L105
  constraint coincident L14.end L104
  constraint perpendicular L14 L104
  constraint tangent L32 A27
  constraint tangent L33 A28
  constraint tangent L35 A29
  constraint tangent L34 A30
  constraint tangent L49 A31
  constraint tangent L49 A32
  constraint tangent L51 A33
  constraint tangent L50 A34
  constraint tangent L57 A35
  constraint tangent L57 A36
  constraint tangent L59 A37
  constraint tangent L58 A38
  constraint tangent L76 A39
  constraint tangent L78 A40
  constraint tangent L79 A41
  constraint tangent L77 A42
  constraint tangent L54 A43
  constraint tangent L54 A44
  constraint tangent L52 A45
  constraint tangent L53 A46
  constraint tangent L90 A47
  constraint tangent L90 A48
  constraint tangent L91 A48
  constraint tangent L91 A49
  constraint tangent L89 A50
  constraint tangent L100 A51
  constraint tangent L101 A52
  constraint tangent L103 A53
  constraint tangent L102 A54
  constraint tangent L93 A55
  constraint tangent L93 A56
  constraint tangent L95 A57
  constraint tangent L94 A58
  constraint tangent L21 A59
  constraint tangent L20 A60
  constraint tangent L22 A60
  constraint tangent L22 A61
  constraint tangent L23 A62
  constraint tangent L64 A63
  constraint tangent L66 A63
  constraint tangent L64 A64
  constraint tangent L65 A65
  constraint tangent L67 A66
  constraint tangent L98 A67
  constraint tangent L98 A68
  constraint tangent L96 A69
  constraint tangent L97 A70
  constraint tangent L70 A71
  constraint tangent L70 A72
  constraint tangent L68 A73
  constraint tangent L69 A74
  constraint tangent L80 A75
  constraint tangent L80 A76
  constraint tangent L82 A76
  constraint tangent L82 A77
  constraint tangent L83 A77
  constraint tangent L83 A78
  constraint tangent L81 A78
  constraint tangent L29 A79
  constraint tangent L29 A80
  constraint tangent L28 A81
  constraint tangent L30 A82
  constraint tangent L37 A83
  constraint tangent L37 A84
  constraint tangent L36 A84
  constraint tangent L36 A85
  constraint tangent L38 A85
  constraint tangent L38 A86
  constraint tangent L39 A86
  constraint tangent L61 A87
  constraint tangent L61 A88
  constraint tangent L60 A88
  constraint tangent L60 A89
  constraint tangent L62 A90
  constraint tangent L40 A91
  constraint tangent L42 A92
  constraint tangent L43 A93
  constraint tangent L41 A93
  constraint tangent L41 A94
  constraint tangent L40 A94
  constraint tangent L44 A95
  constraint tangent L46 A95
  constraint tangent L46 A96
  constraint tangent L47 A96
  constraint tangent L47 A97
  constraint tangent L45 A97
  constraint tangent L45 A98
  constraint tangent L44 A98
  constraint tangent L74 A99
  constraint tangent L75 A99
  constraint tangent L74 A100
  constraint tangent L72 A101
  constraint tangent L73 A102
  constraint tangent L26 A103
  constraint tangent L27 A103
  constraint tangent L26 A104
  constraint tangent L24 A105
  constraint tangent L25 A106
  constraint tangent L86 A107
  constraint tangent L87 A107
  constraint tangent L86 A108
  constraint tangent L84 A109
  constraint tangent L85 A110
  constraint perpendicular L106 L107
  constraint tangent L108 A113
  constraint tangent L107 A113
  constraint tangent L106 A114
  constraint tangent L107 A114
  constraint tangent L108 A115
  constraint perpendicular L104 L109
  constraint perpendicular L109 L110
  constraint tangent L109 A116
  constraint tangent L110 A116
  constraint tangent L110 A117
  constraint tangent A12 L112
  constraint tangent L111 A118
  constraint tangent L112 A118
  constraint concentric A8 A119
  constraint concentric A6 A120
  constraint concentric A23 A121
  constraint concentric A21 A122
  constraint horizontal L113
  constraint perpendicular L113 L114
  constraint parallel L113 L115
  constraint parallel L114 L116
  constraint tangent L116 A123
  constraint tangent L115 A123
  constraint tangent L113 A124
  constraint tangent L116 A124
  constraint tangent L113 A125
  constraint tangent L114 A125
  constraint tangent L114 A126
  constraint tangent L115 A126
  constraint horizontal L117
  constraint perpendicular L117 L118
  constraint parallel L117 L119
  constraint parallel L118 L120
  constraint tangent A130 L120
  constraint tangent L119 A130
  constraint tangent A127 L117
  constraint tangent A127 L120
  constraint tangent L117 A128
  constraint tangent A128 L118
  constraint tangent L118 A129
  constraint tangent A129 L119
  constraint horizontal L121
  constraint perpendicular L121 L122
  constraint parallel L121 L123
  constraint parallel L122 L124
  constraint tangent A134 L124
  constraint tangent L123 A134
  constraint tangent A131 L121
  constraint tangent A131 L124
  constraint tangent L121 A132
  constraint tangent A132 L122
  constraint tangent L122 A133
  constraint tangent A133 L123
  constraint horizontal L125
  constraint perpendicular L125 L126
  constraint parallel L125 L127
  constraint parallel L126 L128
  constraint tangent A138 L128
  constraint tangent L127 A138
  constraint tangent A135 L125
  constraint tangent A135 L128
  constraint tangent L125 A136
  constraint tangent A136 L126
  constraint tangent L126 A137
  constraint tangent A137 L127
  constraint horizontal L129
  constraint perpendicular L129 L130
  constraint parallel L129 L131
  constraint parallel L130 L132
  constraint tangent A142 L132
  constraint tangent L131 A142
  constraint tangent A139 L129
  constraint tangent A139 L132
  constraint tangent L129 A140
  constraint tangent A140 L130
  constraint tangent L130 A141
  constraint tangent A141 L131
  constraint horizontal L133
  constraint perpendicular L133 L134
  constraint parallel L133 L135
  constraint parallel L134 L136
  constraint tangent A146 L136
  constraint tangent L135 A146
  constraint tangent A143 L133
  constraint tangent A143 L136
  constraint tangent L133 A144
  constraint tangent A144 L134
  constraint tangent L134 A145
  constraint tangent A145 L135
  constraint horizontal L137
  constraint perpendicular L137 L138
  constraint parallel L137 L139
  constraint parallel L138 L140
  constraint tangent A150 L140
  constraint tangent L139 A150
  constraint tangent A147 L137
  constraint tangent A147 L140
  constraint tangent L137 A148
  constraint tangent A148 L138
  constraint tangent L138 A149
  constraint tangent A149 L139
  constraint horizontal L141
  constraint perpendicular L141 L142
  constraint parallel L141 L143
  constraint parallel L142 L144
  constraint tangent A154 L144
  constraint tangent L143 A154
  constraint tangent A151 L141
  constraint tangent A151 L144
  constraint tangent L141 A152
  constraint tangent A152 L142
  constraint tangent L142 A153
  constraint tangent A153 L143
  constraint horizontal L145
  constraint perpendicular L145 L146
  constraint parallel L145 L147
  constraint parallel L146 L148
  constraint tangent A158 L148
  constraint tangent L147 A158
  constraint tangent A155 L145
  constraint tangent A155 L148
  constraint tangent L145 A156
  constraint tangent A156 L146
  constraint tangent L146 A157
  constraint tangent A157 L147
  constraint horizontal L157
  constraint perpendicular L157 L158
  constraint parallel L157 L159
  constraint parallel L158 L160
  constraint tangent A170 L160
  constraint tangent L159 A170
  constraint tangent A167 L157
  constraint tangent A167 L160
  constraint tangent L157 A168
  constraint tangent A168 L158
  constraint tangent L158 A169
  constraint tangent A169 L159
  constraint horizontal L153
  constraint perpendicular L153 L154
  constraint parallel L153 L155
  constraint parallel L154 L156
  constraint tangent A166 L156
  constraint tangent L155 A166
  constraint tangent A163 L153
  constraint tangent A163 L156
  constraint tangent L153 A164
  constraint tangent A164 L154
  constraint tangent L154 A165
  constraint tangent A165 L155
  constraint horizontal L149
  constraint perpendicular L149 L150
  constraint parallel L149 L151
  constraint parallel L150 L152
  constraint tangent A162 L152
  constraint tangent L151 A162
  constraint tangent A159 L149
  constraint tangent A159 L152
  constraint tangent L149 A160
  constraint tangent A160 L150
  constraint tangent L150 A161
  constraint tangent A161 L151
  constraint horizontal L169
  constraint perpendicular L169 L170
  constraint parallel L169 L171
  constraint parallel L170 L172
  constraint tangent A182 L172
  constraint tangent L171 A182
  constraint tangent A179 L169
  constraint tangent A179 L172
  constraint tangent L169 A180
  constraint tangent A180 L170
  constraint tangent L170 A181
  constraint tangent A181 L171
  constraint horizontal L165
  constraint perpendicular L165 L166
  constraint parallel L165 L167
  constraint parallel L166 L168
  constraint tangent A178 L168
  constraint tangent L167 A178
  constraint tangent A175 L165
  constraint tangent A175 L168
  constraint tangent L165 A176
  constraint tangent A176 L166
  constraint tangent L166 A177
  constraint tangent A177 L167
  constraint horizontal L161
  constraint perpendicular L161 L162
  constraint parallel L161 L163
  constraint parallel L162 L164
  constraint tangent A174 L164
  constraint tangent L163 A174
  constraint tangent A171 L161
  constraint tangent A171 L164
  constraint tangent L161 A172
  constraint tangent A172 L162
  constraint tangent L162 A173
  constraint tangent A173 L163
  constraint horizontal L173
  constraint perpendicular L173 L174
  constraint parallel L173 L175
  constraint parallel L174 L176
  constraint tangent A186 L176
  constraint tangent L175 A186
  constraint tangent A183 L173
  constraint tangent A183 L176
  constraint tangent L173 A184
  constraint tangent A184 L174
  constraint tangent L174 A185
  constraint tangent A185 L175
  constraint horizontal L189
  constraint perpendicular L189 L190
  constraint parallel L189 L191
  constraint parallel L190 L192
  constraint tangent A202 L192
  constraint tangent L191 A202
  constraint tangent A199 L189
  constraint tangent A199 L192
  constraint tangent L189 A200
  constraint tangent A200 L190
  constraint tangent L190 A201
  constraint tangent A201 L191
  constraint horizontal L185
  constraint perpendicular L185 L186
  constraint parallel L185 L187
  constraint parallel L186 L188
  constraint tangent A198 L188
  constraint tangent L187 A198
  constraint tangent A195 L185
  constraint tangent A195 L188
  constraint tangent L185 A196
  constraint tangent A196 L186
  constraint tangent L186 A197
  constraint tangent A197 L187
  constraint horizontal L181
  constraint perpendicular L181 L182
  constraint parallel L181 L183
  constraint parallel L182 L184
  constraint tangent A194 L184
  constraint tangent L183 A194
  constraint tangent A191 L181
  constraint tangent A191 L184
  constraint tangent L181 A192
  constraint tangent A192 L182
  constraint tangent L182 A193
  constraint tangent A193 L183
  constraint horizontal L177
  constraint perpendicular L177 L178
  constraint parallel L177 L179
  constraint parallel L178 L180
  constraint tangent A190 L180
  constraint tangent L179 A190
  constraint tangent A187 L177
  constraint tangent A187 L180
  constraint tangent L177 A188
  constraint tangent A188 L178
  constraint tangent L178 A189
  constraint tangent A189 L179
  constraint horizontal L193
  constraint perpendicular L193 L194
  constraint parallel L193 L195
  constraint parallel L194 L196
  constraint tangent A206 L196
  constraint tangent L195 A206
  constraint tangent A203 L193
  constraint tangent A203 L196
  constraint tangent L193 A204
  constraint tangent A204 L194
  constraint tangent L194 A205
  constraint tangent A205 L195
  constraint horizontal L197
  constraint perpendicular L197 L198
  constraint parallel L197 L199
  constraint parallel L198 L200
  constraint tangent A210 L200
  constraint tangent L199 A210
  constraint tangent A207 L197
  constraint tangent A207 L200
  constraint tangent L197 A208
  constraint tangent A208 L198
  constraint tangent L198 A209
  constraint tangent A209 L199
  constraint concentric A15 A233
  constraint concentric A14 A234
  constraint concentric A26 A235
  constraint concentric A24 A236
  constraint tangent A233 L226
  constraint tangent A234 L227
  constraint tangent A235 L238
  constraint tangent L238 A236
  constraint tangent L223 A237
  constraint tangent L224 A237
  constraint tangent L223 A238
  constraint tangent L244 A238
  constraint tangent L240 A239
  constraint tangent L241 A239
  constraint tangent L242 A240
  constraint tangent L243 A240
  constraint tangent L244 A241
  constraint tangent L243 A241
  constraint tangent L242 A242
  constraint tangent L241 A242
  constraint tangent L240 A243
  constraint tangent L239 A243
  constraint tangent L225 A244
  constraint tangent L224 A244
  constraint coincident L216 L245.start
  constraint coincident L237 L245.end
  constraint perpendicular L237 L245
  constraint tangent L227 A245
  constraint tangent L228 A245
  constraint tangent L229 A246
  constraint tangent L228 A246
  constraint tangent L229 A247
  constraint tangent L230 A247
  constraint tangent L230 A248
  constraint tangent L231 A248
  constraint tangent L231 A249
  constraint tangent L232 A249
  constraint tangent L232 A250
  constraint tangent L233 A250
  constraint tangent L234 A251
  constraint tangent L235 A251
  constraint tangent L233 A252
  constraint tangent L234 A252
  constraint tangent L236 A253
  constraint tangent L237 A253
  constraint tangent L235 A254
  constraint tangent L236 A254
  constraint coincident L106.end L216
  constraint perpendicular L106 L216
  constraint tangent A115 L246
  constraint horizontal L246
  constraint coincident L215 L246.end
  constraint tangent A117 L247
  constraint perpendicular L215 L247
  constraint coincident L215 L247.end
  constraint coincident L215 L248.start
  constraint perpendicular L238 L248